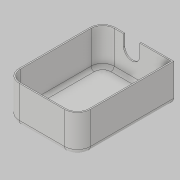
# Autodesk Inventor part: picaseV2
Saved by Autodesk Inventor 2018.3 (Build 223284000, 284)
## iProperties
Created: 2018-03-01
Part Number: picaseV2
Material: Generic
Document SubType Name: Modeling
Designer: mjsi2
Density: 1 g/cm^3
Appearance: Default
Author: mjsi2
Autodesk Inventor part; units mm, degrees
ref_plane "YZ Plane" through (0, 0, 0) normal (1, 0, 0) x (0, 1, 0)
ref_plane "XZ Plane" through (0, 0, 0) normal (0, 1, 0) x (-1, 0, 0)
ref_plane "XY Plane" through (0, 0, 0) normal (0, 0, 1) x (1, 0, 0)
sketch "Sketch1" plane through (0, 0, 0) normal (0, 1, 0) x (-1, 0, 0)
  line L0 (79.7789, 88.5449) -> (79.7789, -61.4551)
  line L1 (79.7789, -61.4551) -> (-31.0159, -61.4551)
  line L2 (-31.0159, -61.4551) -> (-31.0159, 88.5449)
  line L3 (-31.0159, 88.5449) -> (79.7789, 88.5449)
  point P0 (0, 0)
  dimension "d0" = 150
  dimension "d1" = 110.7948
  constraints: 8 end point, 1 parallel, 1 perpendicular
  measures "d0" distance of L0.start L0.end
  measures "d1" distance of L0.end L1.end
extrude "Body" add sketch "Sketch1" along normal blind 58
fillet "Fillet6" radius 20 1 edges at (-79.7789, 29, -61.4551)
fillet "Fillet4" radius 20 1 edges at (-79.7789, 29, 88.5449)
fillet "Fillet2" radius 20 1 edges at (31.0159, 29, 88.5449)
shell "Shell1" thickness 2 removed faces 1 at (-42.8473, 58, 31.8782)
sketch "Sketch6" plane through (31.0159, 0, -61.4551) normal (0, 0, -1) x (-1, 0, 0)
  line L0 (20.28, 18.92) -> (4.4, 18.92)
  line L1 (4.4, 18.92) -> (4.4, 5.42)
  line L2 (4.4, 5.42) -> (20.28, 5.42)
  line L3 (20.28, 5.42) -> (20.28, 18.92)
  line L4 (0, 9.95) -> (4.4, 9.95) construction
  line L5 (0, 0) -> (0, 58) projected
  line L6 (110.7948, 0) -> (0, 0) projected
  line L7 (15.1382, 0) -> (15.1382, 5.42)
  point P0 (20.28, 13.27)
  point P1 (11.2745, 5.42)
  dimension "d38" = 15.88
  dimension "d39" = 13.5
  dimension "d40" = 4.4
  dimension "d97" = 5.42
  constraints: 12 end point, 6 point on line, 2 perpendicular, 1 horizontal, 1 parallel
  measures "d38" distance of L2.start L3.start
  measures "d39" distance of L3.start L0.start
  measures "d40" distance of L4.end L4.start
  measures "d97" distance of L7.start L7.end
extrude "Cut_Ethernet" [suppressed]
sketch "Sketch5" plane through (31.0159, 0, -61.4551) normal (0, 0, -1) x (-1, 0, 0)
  line L0 (24.44, 21.12) -> (37.74, 21.12)
  line L1 (37.74, 21.12) -> (37.74, 5.42)
  line L2 (37.74, 5.42) -> (24.44, 5.42)
  line L3 (24.44, 5.42) -> (24.44, 21.12)
  line L4 (42.44, 10.5231) -> (37.74, 10.5231) construction
  line L5 (28.3152, 0) -> (28.3152, 5.42) construction
  line L6 (20.28, 18.92) -> (20.28, 5.42) projected
  line L7 (20.28, 10.8914) -> (24.44, 10.8914) construction
  line L8 (0, 0) -> (110.7948, 0) projected
  point P0 (31.0159, 0)
  point P1 (24.44, 13.27)
  dimension "d32" = 4.7
  dimension "d33" = 5.42
  dimension "d34" = 13.3
  dimension "d35" = 15.7
  dimension "d62" = 4.16
  constraints: 14 end point, 5 point on line, 2 horizontal, 2 parallel, 2 perpendicular, 1 midpoint, 1 vertical
  measures "d32" distance of L4.start L4.end
  measures "d33" distance of L5.start L5.end
  measures "d34" distance of L1.end L3.start
  measures "d35" distance of L0.end L1.end
  measures "d62" distance of L7.start L7.end
extrude "Cut_USB1" [suppressed]
sketch "Sketch4" plane through (31.0159, 0, -61.4551) normal (0, 0, -1) x (-1, 0, 0)
  line L0 (46.0437, 0) -> (46.0437, 5.42) construction
  line L1 (110.7948, 0) -> (110.7948, 58) projected
  line L2 (42.44, 5.42) -> (55.74, 5.42)
  line L3 (55.74, 5.42) -> (55.74, 21.12)
  line L4 (55.74, 21.12) -> (42.44, 21.12)
  line L5 (42.44, 21.12) -> (42.44, 5.42)
  line L6 (24.44, 21.12) -> (37.74, 21.12)
  line L7 (37.74, 21.12) -> (37.74, 5.42)
  line L8 (37.74, 5.42) -> (24.44, 5.42)
  line L9 (24.44, 5.42) -> (24.44, 21.12)
  line L10 (42.44, 10.5231) -> (37.74, 10.5231) construction
  line L11 (53.709, 2.22) -> (53.709, 5.42) construction
  line L12 (24.44, 13.27) -> (20.28, 13.27) construction
  line L13 (20.28, 18.92) -> (4.4, 18.92)
  line L14 (4.4, 18.92) -> (4.4, 5.42)
  line L15 (4.4, 5.42) -> (20.28, 5.42)
  line L16 (20.28, 5.42) -> (20.28, 18.92)
  line L17 (36.6745, 2.22) -> (36.6745, 5.42) construction
  line L18 (0, 0) -> (0, 58) projected
  line L19 (31.09, 0) -> (31.09, 5.42) construction
  line L20 (4.4, 5.42) -> (4.4, 18.92) projected
  line L21 (0, 0) -> (110.7948, 0) projected
  line L22 (13.4846, 5.42) -> (13.4846, 0) construction
  point P0 (31.0159, 0)
  point P1 (4.4, 12.17)
  dimension "d16" = 5.42
  dimension "d18" = 13.3
  dimension "d19" = 15.7
  dimension "d20" = 4.7
  dimension "d21" = 3.2
  dimension "d22" = 13.3
  dimension "d23" = 15.7
  dimension "d24" = 4.16
  dimension "d25" = 15.88
  dimension "d26" = 13.5
  dimension "d27" = 3.2
  dimension "d29" = 5.42
  dimension "d98" = 5.42
  constraints: 38 end point, 7 point on line, 6 parallel, 5 vertical, 4 horizontal, 4 midpoint, 3 perpendicular, 4 other
  measures "d16" distance of L0.start L0.end
  measures "d18" distance of L2.start L2.end
  measures "d19" distance of L4.end L2.start
  measures "d20" distance of L10.start L10.end
  measures "d21" distance of L11.start L11.end
  measures "d22" distance of L7.end L8.end
  measures "d23" distance of L6.end L7.end
  measures "d24" distance of L12.start L12.end
  measures "d25" distance of L14.end L15.end
  measures "d26" distance of L15.end L13.start
  measures "d27" distance of L17.start L17.end
  measures "d29" distance of L19.end L19.start
  measures "d98" distance of L22.start L22.end
extrude "Cut_USB2" [suppressed]
fillet "Fillet10" radius 5 7 edges at (-77.7789, 2, 13.5449) (-72.5068, 2, 81.2728) (-24.3815, 2, 86.5449) (23.7438, 2, 81.2728) (29.0159, 2, 4.5449) (-72.5068, 2, -54.183) (-15.3815, 2, -59.4551)
fillet "Fillet9" radius 8 7 edges at (-14.3815, 0, -61.4551) (-73.921, 0, -55.5972) (-79.7789, 0, 13.5449) (-73.921, 0, 82.687) (-24.3815, 0, 88.5449) (25.158, 0, 82.687) (31.0159, 0, 3.5449)
sketch "Sketch13" plane through (-59.7789, 0, -61.4551) normal (0, 0, -1) x (-1, 0, 0)
  circle A0 centre (-59.7048, 47.625) radius 4.1 construction
  line L0 (-66.3548, 21.12) -> (-53.0548, 21.12) projected
  line L1 (-59.7048, 21.12) -> (-59.7048, 61.9125) construction
  line L2 (-79.7048, 53.975) -> (-39.7048, 53.975)
  line L3 (-39.7048, 53.975) -> (-39.7048, 25.4)
  line L4 (-39.7048, 25.4) -> (-79.7048, 25.4) construction
  line L5 (-79.7048, 25.4) -> (-79.7048, 53.975)
  line L6 (-79.7048, 39.6875) -> (-39.7048, 39.6875) construction
  line L7 (-79.7048, 42.1875) -> (-39.7048, 42.1875)
  line L8 (-39.7048, 42.1875) -> (-39.7048, 37.1875)
  line L9 (-39.7048, 37.1875) -> (-79.7048, 37.1875) construction
  line L10 (-79.7048, 37.1875) -> (-79.7048, 42.1875)
  line L11 (-74.6125, 42.1875) -> (-74.6125, 37.1875) construction
  line L12 (-79.7048, 42.1875) -> (-79.7048, 53.975)
  line L13 (-39.7048, 53.975) -> (-39.7048, 42.1875)
  point P0 (-59.7789, 0)
  point P1 (-59.7048, 53.975)
  dimension "d93" = 8.2
  dimension "d96" = 40
  dimension "d104" = 5
  dimension "d105" = 28.575
  constraints: 26 end point, 6 midpoint, 5 parallel, 4 perpendicular, 4 point on line, 2 horizontal, 1 centre point, 1 vertical
  measures "d93" diameter of A0
  measures "d96" distance of L2.start L2.end
  measures "d104" distance of L11.start L11.end
  measures "d105" distance of L2.end L3.end
extrude "Extrusion13" [suppressed]
sketch "Sketch15" plane through (31.0159, 58, -61.4551) normal (0, 0, -1) x (-1, 0, 0)
  circle A0 centre (31.09, -10.375) radius 4.1 construction
  line L0 (24.44, -36.88) -> (37.74, -36.88)
  line L1 (31.09, -36.88) -> (31.09, 3.9125) construction
  line L2 (11.09, -4.025) -> (51.09, -4.025) construction
  line L3 (51.09, -4.025) -> (51.09, -32.6) construction
  line L4 (51.09, -32.6) -> (11.09, -32.6)
  line L5 (11.09, -32.6) -> (11.09, -4.025) construction
  line L6 (11.09, -18.3125) -> (51.09, -18.3125) construction
  line L7 (11.09, -15.8125) -> (51.09, -15.8125) construction
  line L8 (51.09, -15.8125) -> (51.09, -20.8125)
  line L9 (51.09, -20.8125) -> (11.09, -20.8125)
  line L10 (11.09, -20.8125) -> (11.09, -15.8125)
  line L11 (16.1823, -15.8125) -> (16.1823, -20.8125) construction
  line L12 (51.09, -4.025) -> (11.1125, -4.025) construction
  line L13 (11.09, -20.8125) -> (11.09, -32.6)
  line L14 (51.09, -32.6) -> (51.09, -20.8125)
  point P0 (31.0159, -58)
  point P1 (-59.7789, 0)
  point P2 (31.09, -4.025)
  dimension "d106" = 8.2
  dimension "d107" = 40
  dimension "d108" = 5
  dimension "d109" = 28.575
  constraints: 30 end point, 6 midpoint, 5 parallel, 4 perpendicular, 4 point on line, 3 horizontal, 1 centre point, 1 vertical
  measures "d106" diameter of A0
  measures "d107" distance of L2.start L2.end
  measures "d108" distance of L11.start L11.end
  measures "d109" distance of L2.end L3.end
extrude "Extrusion14" [suppressed]
sketch "Sketch17" plane through (31.0159, 58, -61.4551) normal (0, 0, -1) x (-1, 0, 0)
  arc A0 (50.8, -17.4625) -> (76.2, -17.4625) centre (63.5, -17.4625) ccw
  line L0 (20, 0) -> (90.7948, 0) projected
  line L1 (50.8, -17.4625) -> (76.2, -17.4625) construction
  line L2 (76.2, -17.4625) -> (76.2, 0)
  line L3 (76.2, 0) -> (72.7075, 0)
  line L4 (50.8, 0) -> (50.8, -17.4625)
  line L5 (0, 0) -> (90.7948, 0) projected
  point P0 (31.0159, -58)
  dimension "d117" = 25.4
  dimension "d124" = 25.4
  constraints: 8 end point, 2 parallel, 2 point on circle, 2 point on line, 1 centre point, 1 horizontal, 1 midpoint, 1 perpendicular
  measures "d117" diameter of A0
  measures "d124" distance of L1.start L1.end
extrude "Extrusion16" cut sketch "Sketch17" against normal blind 2
body "Solid1"
